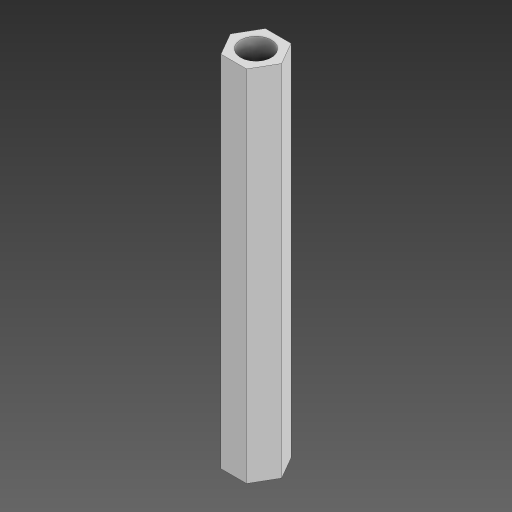
# Autodesk Inventor part: Stoics
Saved by Autodesk Inventor 2023 (Build 270158000, 158)
## iProperties
Created: 2025-06-30
Part Number: Stoics
Material: Типовые
Document SubType Name: Modeling
Designer: daa
Density: 1 g/cm^3
Appearance: По умолчанию
Author: daa
Autodesk Inventor part; units mm, degrees
ref_plane "YZ Plane" through (0, 0, 0) normal (1, 0, 0) x (0, 1, 0)
ref_plane "XZ Plane" through (0, 0, 0) normal (0, 1, 0) x (-1, 0, 0)
ref_plane "XY Plane" through (0, 0, 0) normal (0, 0, 1) x (1, 0, 0)
sketch "Эскиз1" plane through (0, 0, 0) normal (0, 1, 0) x (-1, 0, 0)
  circle A0 centre (0, 0) radius 2.5
  dimension "d0" = 5
  constraints: 1 centre point, 1 coincident
  measures "d0" diameter of A0
extrude "Выдавливание1" add sketch "Эскиз1" along normal blind 35
sketch "Эскиз2" plane through (0, 35, 0) normal (0, 1, 0) x (1, 0, 0)
  circle A0 centre (0, 0) radius 2.5 projected
  line L0 (2.5, 0) -> (1.25, -2.1651)
  line L1 (1.25, -2.1651) -> (-1.25, -2.1651)
  line L2 (-1.25, -2.1651) -> (-2.5, 0)
  line L3 (-2.5, 0) -> (-1.25, 2.1651)
  line L4 (-1.25, 2.1651) -> (1.25, 2.1651)
  line L5 (1.25, 2.1651) -> (2.5, 0)
  point P0 (1.25, 2.1651)
  point P1 (1.25, 2.1651)
  point P2 (-2.5, 0)
  point P3 (-2.5, 0)
  point P4 (-1.25, -2.1651)
  point P5 (-1.25, -2.1651)
  constraints: 12 end point, 1 coincident, 15 other
extrude "Выдавливание2" cut sketch "Эскиз2" against normal through all contours L5 A0 | A0 L0 | L4 A0 | A0 L1 | L3 A0 | A0 L2
sketch "Эскиз3" plane through (0, 0, 0) normal (0, -1, 0) x (1, 0, 0)
  circle A0 centre (0, 0) radius 1.5
  dimension "d5" = 3
  constraints: 1 centre point, 1 coincident
  measures "d5" diameter of A0
extrude "Выдавливание3" cut sketch "Эскиз3" against normal through all
